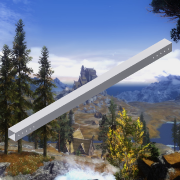
# Autodesk Inventor part: C24R2_TK_ShooterPivotStock
Saved by Autodesk Inventor 2015 SP1 (Build 190203100, 203)
## iProperties
Created: 2016-01-29
Part Number: C24R2_TK_ShooterPivotStock
Material: Generic
Document SubType Name: Modeling
Designer: TheeTimatahee
Density: 1 g/cm^3
Appearance: Default
Mass: 492.374 g
Surface Area: 1181.5 cm^2
Volume: 182.361 cm^3
Author: TheeTimatahee
Autodesk Inventor part; units mm, degrees
ref_plane "YZ Plane" through (0, 0, 0) normal (1, 0, 0) x (0, 1, 0)
ref_plane "XZ Plane" through (0, 0, 0) normal (0, 1, 0) x (-1, 0, 0)
sketch "Sketch1" plane through (0, 0, 0) normal (0, 0, 1) x (1, 0, 0)
  line L0 (-12.7, -12.7) -> (12.7, -12.7)
  line L1 (12.7, -12.7) -> (12.7, 12.7)
  line L2 (12.7, 12.7) -> (-12.7, 12.7)
  line L3 (-12.7, 12.7) -> (-12.7, -12.7)
  line L4 (-12.7, -12.7) -> (12.7, 12.7) construction
  line L5 (12.7, -12.7) -> (-12.7, 12.7) construction
  line L6 (9.525, -9.525) -> (-9.525, -9.525)
  line L7 (-9.525, -9.525) -> (-9.525, 9.525)
  line L8 (-9.525, 9.525) -> (9.525, 9.525)
  line L9 (9.525, 9.525) -> (9.525, -9.525)
  line L10 (9.525, -9.525) -> (-9.525, 9.525) construction
  line L11 (-9.525, -9.525) -> (9.525, 9.525) construction
  point P0 (0, 0)
  dimension "d0" = 25.4
  dimension "d1" = 25.4
  dimension "d6" = 3.175
  dimension "d7" = 3.175
  constraints: 24 end point, 4 midpoint, 4 parallel, 2 horizontal, 2 perpendicular
  measures "d0" distance of L2.end L1.end
  measures "d1" distance of L0.end L1.end
  measures "d6" distance between parallel lines of L2 L8
  measures "d7" distance between parallel lines of L3 L7
extrude "Extrusion1" add sketch "Sketch1" along normal blind 660.4
sketch "Sketch2" plane through (-12.7, -12.7, 0) normal (-1, 0, 0) x (0, 0, 1)
  line L0 (95.377, -0.127) -> (131.064, -0.127) projected
  line L1 (131.064, -0.127) -> (133.223, 2.032) projected
  line L2 (133.223, 2.032) -> (133.223, 23.114) projected
  line L3 (133.223, 23.114) -> (131.064, 25.273) projected
  line L4 (131.064, 25.273) -> (65.786, 25.273) projected
  line L5 (65.786, 25.273) -> (63.627, 23.114) projected
  line L6 (63.627, 23.114) -> (63.627, -42.164) projected
  line L7 (63.627, -42.164) -> (65.786, -44.323) projected
  line L8 (65.786, -44.323) -> (86.868, -44.323) projected
  line L9 (86.868, -44.323) -> (89.027, -42.164) projected
  line L10 (89.027, -6.477) -> (89.027, -42.164) projected
  arc A0 (95.377, -0.127) -> (89.027, -6.477) centre (95.377, -6.477) ccw projected
  circle A1 centre (127, 12.7) radius 2.0701 projected
  circle A2 centre (76.2, -25.4) radius 2.0701 projected
  circle A3 centre (76.2, 0) radius 2.0701 projected
  circle A4 centre (101.6, 12.7) radius 2.0701 projected
  circle A5 centre (76.2, 12.7) radius 2.0701 projected
  circle A6 centre (88.9, 12.7) radius 2.0701 projected
  circle A7 centre (114.3, 12.7) radius 2.0701 projected
  circle A8 centre (76.2, -12.7) radius 2.0701 projected
  circle A9 centre (76.2, -38.1) radius 2.0701 projected
  line L11 (527.177, 2.032) -> (527.177, 23.114) projected
  line L12 (527.177, 2.032) -> (529.336, -0.127) projected
  line L13 (565.023, -0.127) -> (529.336, -0.127) projected
  arc A10 (571.373, -6.477) -> (565.023, -0.127) centre (565.023, -6.477) ccw projected
  line L14 (571.373, -6.477) -> (571.373, -42.164) projected
  line L15 (571.373, -42.164) -> (573.532, -44.323) projected
  line L16 (594.614, -44.323) -> (573.532, -44.323) projected
  line L17 (594.614, -44.323) -> (596.773, -42.164) projected
  line L18 (596.773, 23.114) -> (596.773, -42.164) projected
  line L19 (596.773, 23.114) -> (594.614, 25.273) projected
  line L20 (529.336, 25.273) -> (594.614, 25.273) projected
  line L21 (529.336, 25.273) -> (527.177, 23.114) projected
  circle A11 centre (533.4, 12.7) radius 2.0701 projected
  circle A12 centre (584.2, -25.4) radius 2.0701 projected
  circle A13 centre (584.2, 0) radius 2.0701 projected
  circle A14 centre (558.8, 12.7) radius 2.0701 projected
  circle A15 centre (584.2, 12.7) radius 2.0701 projected
  circle A16 centre (571.5, 12.7) radius 2.0701 projected
  circle A17 centre (546.1, 12.7) radius 2.0701 projected
  circle A18 centre (584.2, -12.7) radius 2.0701 projected
  circle A19 centre (584.2, -38.1) radius 2.0701 projected
  point P0 (0, 12.7)
hole "Hole1" at (-12.7, 0, 127) at (-12.7, 0, 114.3) at (-12.7, 0, 101.6) at (-12.7, 0, 88.9) at (-12.7, 0, 76.2) at (-12.7, 0, 584.2) at (-12.7, 0, 571.5) at (-12.7, 0, 558.8) at (-12.7, 0, 546.1) at (-12.7, 0, 533.4) direction (1, 0, 0) diameter 4.1402 end through all
sketch "Sketch7" plane through (0, 0, 0) normal (0, 0, -1) x (-1, 0, 0)
  line L0 (9.525, 9.525) -> (9.525, -9.525) projected
  line L1 (9.525, -9.525) -> (-9.525, -9.525) projected
  line L2 (-9.525, -9.525) -> (-9.525, 9.525) projected
  line L3 (-9.525, 9.525) -> (9.525, 9.525) projected
  line L4 (-12.7, 12.7) -> (12.7, 12.7) projected
  line L5 (-11.1125, -11.1125) -> (11.1125, -11.1125)
  line L6 (11.1125, -11.1125) -> (11.1125, 11.1125)
  line L7 (11.1125, 11.1125) -> (-11.1125, 11.1125)
  line L8 (-11.1125, 11.1125) -> (-11.1125, -11.1125)
  line L9 (-11.1125, -11.1125) -> (11.1125, 11.1125) construction
  line L10 (11.1125, -11.1125) -> (-11.1125, 11.1125) construction
  point P0 (0, 0)
  dimension "d33" = 1.5875
  constraints: 12 end point, 2 midpoint, 2 parallel, 2 perpendicular, 1 horizontal
  measures "d33" distance between parallel lines of L4 L7
extrude "Extrusion5" cut sketch "Sketch7" against normal through all
ref_plane "Work Plane1" through (17.4625, -12.7, 0) normal (1, 0, 0) x (0, 0, -1)
sketch "Sketch9" plane through (12.7, -12.7, 0) normal (1, 0, 0) x (0, 0, -1)
  line L0 (-660.4, 25.4) -> (-596.9, 25.4)
  line L1 (-596.9, 25.4) -> (-596.9, 0)
  line L2 (-596.9, 0) -> (-660.4, 0)
  line L3 (-660.4, 0) -> (-660.4, 25.4)
  line L4 (0, 25.4) -> (-63.5, 25.4)
  line L5 (-63.5, 25.4) -> (-63.5, 0)
  line L6 (-63.5, 0) -> (0, 0)
  line L7 (0, 0) -> (0, 25.4)
  line L8 (0, 0) -> (-660.4, 0) projected
  point P0 (0, 12.7)
  dimension "d42" = 63.5
  dimension "d43" = 63.5
  constraints: 16 end point, 4 parallel, 2 collinear, 2 horizontal, 2 perpendicular
  measures "d42" distance between parallel lines of L5 L7
  measures "d43" distance between parallel lines of L3 L1
extrude "Extrusion7" cut sketch "Sketch9" against normal through all
body "Solid1"
